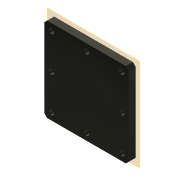
# Autodesk Inventor part: 00_XY_stage-CHUO_SEIKI_LD-647-R1-Bottom
Saved by Autodesk Inventor 2022 (Build 260153000, 153)
## iProperties
Created: 2019-05-02
Part Number: 00_XY_stage-CHUO_SEIKI_LD-647-R1-Bottom
Material: Generic
Document SubType Name: Modeling
Designer: diederichbenedict
Density: 1 g/cm^3
Appearance: Gunmetal
Author: diederichbenedict
Autodesk Inventor part; units mm, degrees
ref_plane "YZ Plane" through (0, 0, 0) normal (1, 0, 0) x (0, 1, 0)
ref_plane "XZ Plane" through (0, 0, 0) normal (0, 1, 0) x (-1, 0, 0)
ref_plane "XY Plane" through (0, 0, 0) normal (0, 0, 1) x (1, 0, 0)
ref_plane "Work Plane1" through (0, 0, 0) normal (0, 0, 1) x (1, 0, 0)
sketch "Sketch1" plane through (0, 0, 0) normal (0, 0, 1) x (1, 0, 0)
  line L0 (-28, 30) -> (-30, 28) projected
  line L1 (-30, 28) -> (-30, -28) projected
  line L2 (-30, -28) -> (-28, -30) projected
  line L3 (-28, -30) -> (28, -30) projected
  line L4 (28, -30) -> (30, -28) projected
  line L5 (30, -28) -> (30, -17.7934) projected
  line L6 (30, 28) -> (28, 30) projected
  line L7 (28, 30) -> (17.7934, 30) projected
  line L8 (-25, -25) -> (25, -25) construction
  line L9 (25, -25) -> (25, 25) construction
  line L10 (25, 25) -> (-25, 25) construction
  line L11 (-25, 25) -> (-25, -25) construction
  line L12 (-25, -25) -> (25, 25) construction
  line L13 (25, -25) -> (-25, 25) construction
  line L14 (30, -17.7934) -> (44, -17.7934) projected
  line L15 (44, -9.0511) -> (44, -17.7934) projected
  line L16 (30, -9.0511) -> (44, -9.0511) construction
  line L17 (30, -9.0511) -> (30, 8.3051) projected
  line L18 (30, 8.3051) -> (44, 8.3051) projected
  line L19 (44, 19.2331) -> (44, 8.3051) projected
  line L20 (30, 19.2331) -> (44, 19.2331) construction
  line L21 (30, 28) -> (30, -28) projected
  line L22 (17.7934, 30) -> (17.7934, 44) projected
  line L23 (9.0511, 44) -> (17.7934, 44) projected
  line L24 (9.0511, 30) -> (9.0511, 44) construction
  line L25 (-8.3051, 30) -> (-8.3051, 44) projected
  line L26 (-19.2331, 44) -> (-8.3051, 44) projected
  line L27 (-19.2331, 30) -> (-19.2331, 44) construction
  line L28 (-19.2331, 30) -> (-28, 30) projected
  line L29 (30, 19.2331) -> (30, 28) projected
  line L30 (9.0511, 30) -> (-8.3051, 30) projected
  line L31 (-28, 30) -> (28, 30) projected
  line L32 (25, 0) -> (-25, 0)
  point P0 (0, 0)
  dimension "d0" = 50
  dimension "d1" = 50
  constraints: 14 end point, 4 midpoint, 2 parallel, 1 horizontal, 1 perpendicular
  measures "d0" distance of L10.end L9.end
  measures "d1" distance of L9.end L8.end
extrude "Extrusion1" add sketch "Sketch1" along normal blind 6
sketch "Sketch2" plane through (0, 0, 6) normal (0, 0, 1) x (1, 0, 0)
  line L0 (-25, -25) -> (25, -25)
  line L1 (25, -25) -> (25, 25)
  line L2 (25, 25) -> (-25, 25)
  line L3 (-25, 25) -> (-25, -25)
  line L4 (-25, -25) -> (25, 25) construction
  line L5 (25, -25) -> (-25, 25) construction
  point P0 (0, 0)
  point P1 (25, 0)
  point P2 (-25, 0)
  point P3 (0, 25)
  point P4 (0, -25)
  dimension "d4" = 50
  dimension "d5" = 50
  constraints: 12 end point, 6 midpoint, 2 parallel, 1 horizontal, 1 perpendicular
  measures "d4" distance of L2.end L1.end
  measures "d5" distance of L1.end L0.end
hole "Hole1" at (25, 25, 6) at (25, -25, 6) at (-25, -25, 6) at (-25, 25, 6) at (-25, 0, 6) at (25, 0, 6) at (0, 25, 6) at (0, -25, 6) direction (0, 0, -1) diameter 3.9 depth 10 tip angle 118
body "Solid1"
